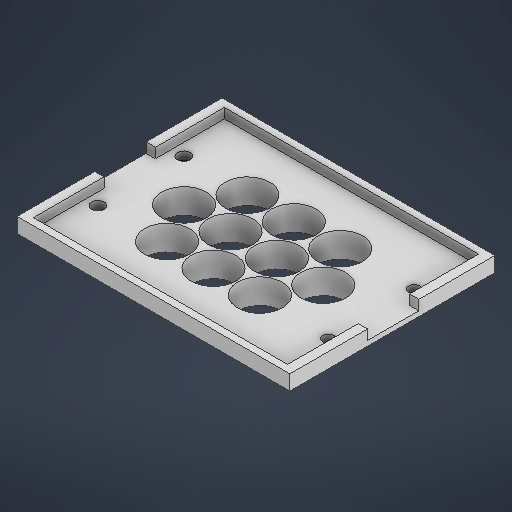
# Autodesk Inventor part: CELLCASE26650
Saved by Autodesk Inventor 2025.2 (Build 292293000, 293)
## iProperties
Created: 2025-01-16
Part Number: CELLCASE26650
Material: Generic
Document SubType Name: Modeling
Designer: cbast
Density: 1 g/cm^3
Appearance: Default
Author: cbast
## iProperties of the stored document CELLCASE26650_3DPrint.ipt
Created: 2025-01-31
Part Number: CELLCASE26650_3DPrint
Material: Generic
Document SubType Name: Modeling
Designer: cbast
Density: 1 g/cm^3
Appearance: Default
Author: cbast
Autodesk Inventor part; units mm, degrees
ref_plane "YZ Plane" through (0, 0, 0) normal (1, 0, 0) x (0, 1, 0)
ref_plane "XZ Plane" through (0, 0, 0) normal (0, 1, 0) x (-1, 0, 0)
ref_plane "XY Plane" through (0, 0, 0) normal (0, 0, 1) x (1, 0, 0)
sketch "Sketch1" plane through (0, 0, 0) normal (0, 1, 0) x (-1, 0, 0)
  circle A0 centre (0, 0) radius 13.5
  circle A1 centre (0, 0) radius 14.5 construction
  circle A2 centre (28, 0) radius 13.5
  circle A3 centre (28, 0) radius 14.5 construction
  circle A4 centre (56, 0) radius 13.5
  circle A5 centre (56, 0) radius 14.5 construction
  circle A6 centre (84, 0) radius 13.5
  circle A7 centre (84, 0) radius 14.5 construction
  circle A8 centre (14, 24.2487) radius 13.5
  circle A9 centre (42, 24.2487) radius 13.5
  circle A10 centre (70, 24.2487) radius 13.5
  circle A11 centre (70, -24.2487) radius 13.5
  circle A12 centre (42, -24.2487) radius 13.5
  circle A13 centre (14, -24.2487) radius 13.5
  line L0 (84, 0) -> (56, 0) construction
  circle A14 centre (14, 24.2487) radius 14.5 construction
  circle A15 centre (42, 24.2487) radius 14.5 construction
  circle A16 centre (70, 24.2487) radius 14.5 construction
  circle A17 centre (70, -24.2487) radius 14.5 construction
  circle A18 centre (42, -24.2487) radius 14.5 construction
  circle A19 centre (14, -24.2487) radius 14.5 construction
  circle A20 centre (0, 0) radius 15.5 construction
  circle A21 centre (14, 24.2487) radius 15.5 construction
  circle A22 centre (42, 24.2487) radius 15.5 construction
  circle A23 centre (70, 24.2487) radius 15.5 construction
  circle A24 centre (70, -24.2487) radius 15.5 construction
  circle A25 centre (42, -24.2487) radius 15.5 construction
  circle A26 centre (14, -24.2487) radius 15.5 construction
  arc A27 (1.2391, 15.4504) -> (1.2391, -15.4504) centre (0, 0) ccw
  arc A28 (28, 30.9008) -> (1.2391, 15.4504) centre (14, 24.2487) ccw
  arc A29 (56, 30.9008) -> (28, 30.9008) centre (42, 24.2487) ccw
  line L1 (70, 24.2487) -> (14, 24.2487) construction
  line L2 (14, 24.2487) -> (14, -24.2487) construction
  line L3 (14, -24.2487) -> (70, -24.2487) construction
  line L4 (70, -24.2487) -> (70, 24.2487) construction
  circle A30 centre (84, 0) radius 15.5 construction
  arc A31 (82.7609, 15.4504) -> (56, 30.9008) centre (70, 24.2487) ccw
  arc A32 (82.7609, -15.4504) -> (82.7609, 15.4504) centre (84, 0) ccw
  arc A33 (56, -30.9008) -> (82.7609, -15.4504) centre (70, -24.2487) ccw
  arc A34 (28, -30.9008) -> (56, -30.9008) centre (42, -24.2487) ccw
  arc A35 (1.2391, -15.4504) -> (28, -30.9008) centre (14, -24.2487) ccw
  dimension "d0" = 27
  dimension "d1" = 29
  dimension "d2" = 27
  dimension "d3" = 29
  dimension "d4" = 27
  dimension "d5" = 29
  dimension "d6" = 27
  dimension "d7" = 29
  dimension "d8" = 27
  dimension "d9" = 27
  dimension "d10" = 27
  dimension "d11" = 27
  dimension "d12" = 27
  dimension "d13" = 27
  dimension "d14" = 29
  dimension "d15" = 29
  dimension "d16" = 29
  dimension "d17" = 29
  dimension "d18" = 29
  dimension "d19" = 29
  dimension "d20" = 31
  dimension "d21" = 31
  dimension "d22" = 31
  dimension "d23" = 31
  dimension "d24" = 31
  dimension "d25" = 31
  dimension "d26" = 31
  dimension "d27" = 31
  constraints: 36 centre point, 32 point on circle, 27 coincident, 15 tangent, 10 end point, 2 horizontal, 1 perpendicular
  measures "d0" diameter of A0
  measures "d1" diameter of A1
  measures "d2" diameter of A2
  measures "d3" diameter of A3
  measures "d4" diameter of A4
  measures "d5" diameter of A5
  measures "d6" diameter of A6
  measures "d7" diameter of A7
  measures "d8" diameter of A8
  measures "d9" diameter of A9
  measures "d10" diameter of A10
  measures "d11" diameter of A11
  measures "d12" diameter of A12
  measures "d13" diameter of A13
  measures "d14" diameter of A14
  measures "d15" diameter of A15
  measures "d16" diameter of A16
  measures "d17" diameter of A17
  measures "d18" diameter of A18
  measures "d19" diameter of A19
  measures "d20" diameter of A20
  measures "d21" diameter of A21
  measures "d22" diameter of A22
  measures "d23" diameter of A23
  measures "d24" diameter of A24
  measures "d25" diameter of A25
  measures "d26" diameter of A26
  measures "d27" diameter of A30
extrude "Extrusion1" add sketch "Sketch1" along normal blind 15
sketch "Sketch2" plane through (0, 15, 0) normal (0, 1, 0) x (1, 0, 0)
  arc A0 (-1.2391, 15.4504) -> (-28, 30.9008) centre (-14, 24.2487) ccw projected
  arc A1 (-28, 30.9008) -> (-56, 30.9008) centre (-42, 24.2487) ccw projected
  arc A2 (-56, 30.9008) -> (-82.7609, 15.4504) centre (-70, 24.2487) ccw projected
  arc A3 (-82.7609, 15.4504) -> (-82.7609, -15.4504) centre (-84, 0) ccw projected
  arc A4 (-82.7609, -15.4504) -> (-56, -30.9008) centre (-70, -24.2487) ccw projected
  arc A5 (-56, -30.9008) -> (-28, -30.9008) centre (-42, -24.2487) ccw projected
  arc A6 (-28, -30.9008) -> (-1.2391, -15.4504) centre (-14, -24.2487) ccw projected
  arc A7 (-1.2391, -15.4504) -> (-1.2391, 15.4504) centre (0, 0) ccw projected
  circle A8 centre (-14, 24.2487) radius 13.5 projected
  circle A9 centre (-42, 24.2487) radius 13.5 projected
  circle A10 centre (-70, 24.2487) radius 13.5 projected
  circle A11 centre (-70, -24.2487) radius 13.5 projected
  circle A12 centre (-42, -24.2487) radius 13.5 projected
  circle A13 centre (-14, -24.2487) radius 13.5 projected
  circle A14 centre (-84, 0) radius 13.5 projected
  circle A15 centre (-56, 0) radius 13.5 projected
  circle A16 centre (-28, 0) radius 13.5 projected
  circle A17 centre (0, 0) radius 13.5 projected
  line L0 (-116.8, -58.15) -> (36.6, -58.15)
  line L1 (36.6, -58.15) -> (36.6, 57.15)
  line L2 (36.6, 57.15) -> (-116.8, 57.15)
  line L3 (-116.8, 57.15) -> (-116.8, -58.15)
  line L4 (-116.8, -58.15) -> (36.6, 57.15) construction
  line L5 (36.6, -58.15) -> (-116.8, 57.15) construction
  arc A18 (-82.7609, 15.4504) -> (-82.7609, -15.4504) centre (-84, 0) ccw
  arc A19 (-56, 30.9008) -> (-82.7609, 15.4504) centre (-70, 24.2487) ccw
  arc A20 (-28, 30.9008) -> (-56, 30.9008) centre (-42, 24.2487) ccw
  arc A21 (-1.2391, 15.4504) -> (-28, 30.9008) centre (-14, 24.2487) ccw
  arc A22 (-1.2391, -15.4504) -> (-1.2391, 15.4504) centre (0, 0) ccw
  arc A23 (-28, -30.9008) -> (-1.2391, -15.4504) centre (-14, -24.2487) ccw
  arc A24 (-56, -30.9008) -> (-28, -30.9008) centre (-42, -24.2487) ccw
  arc A25 (-82.7609, -15.4504) -> (-56, -30.9008) centre (-70, -24.2487) ccw
  point P0 (-40.1, -0.5)
  dimension "d30" = 153.4
  dimension "d31" = 115.3
  constraints: 16 point on circle, 12 end point, 8 centre point, 8 coincident, 2 midpoint, 2 parallel, 1 horizontal, 1 perpendicular
  measures "d30" distance of L2.end L1.end
  measures "d31" distance of L1.end L0.end
extrude "Extrusion2" add sketch "Sketch2" against normal blind 5 contours L3 L2 L1 L0
sketch "Sketch3" plane through (0, 15, 0) normal (0, 1, 0) x (1, 0, 0)
  line L0 (36.6, -58.15) -> (36.6, 57.15) projected
  line L1 (36.6, 57.15) -> (-116.8, 57.15) projected
  line L2 (-116.8, 57.15) -> (-116.8, -58.15) projected
  line L3 (-116.8, -58.15) -> (36.6, -58.15) projected
  circle A0 centre (-14, 24.2487) radius 13.5 projected
  circle A1 centre (-42, 24.2487) radius 13.5 projected
  circle A2 centre (-70, 24.2487) radius 13.5 projected
  circle A3 centre (-70, -24.2487) radius 13.5 projected
  circle A4 centre (-42, -24.2487) radius 13.5 projected
  circle A5 centre (-14, -24.2487) radius 13.5 projected
  circle A6 centre (-84, 0) radius 13.5 projected
  circle A7 centre (-56, 0) radius 13.5 projected
  circle A8 centre (-28, 0) radius 13.5 projected
  circle A9 centre (0, 0) radius 13.5 projected
  line L4 (-122.402, -62.3606) -> (42.202, -62.3606)
  line L5 (42.202, -62.3606) -> (42.202, 61.3606)
  line L6 (42.202, 61.3606) -> (-122.402, 61.3606)
  line L7 (-122.402, 61.3606) -> (-122.402, -62.3606)
  line L8 (-122.402, -62.3606) -> (42.202, 61.3606) construction
  line L9 (42.202, -62.3606) -> (-122.402, 61.3606) construction
  line L10 (-116.8, -58.15) -> (36.6, -58.15)
  line L11 (36.6, -58.15) -> (36.6, 57.15)
  line L12 (36.6, 57.15) -> (-116.8, 57.15)
  line L13 (-116.8, 57.15) -> (-116.8, -58.15)
  line L14 (-116.8, -58.15) -> (36.6, 57.15) construction
  line L15 (36.6, -58.15) -> (-116.8, 57.15) construction
  point P0 (-40.1, -0.5)
  constraints: 24 end point, 4 midpoint, 4 parallel, 4 point on line, 2 horizontal, 2 perpendicular
extrude "Extrusion3" add sketch "Sketch3" along normal blind 6 and the other way blind 3 contours L7 L6 L5 L4
sketch "Sketch4" plane through (0, 15, 0) normal (0, 1, 0) x (1, 0, 0)
  line L0 (36.6, -58.15) -> (36.6, 57.15) construction
  line L1 (36.6, 57.15) -> (-116.8, 57.15) construction
  line L2 (-116.8, 57.15) -> (-116.8, -58.15) construction
  line L3 (-116.8, -58.15) -> (36.6, -58.15) construction
  circle A0 centre (-14, 24.2487) radius 13.5 construction
  circle A1 centre (-42, 24.2487) radius 13.5 construction
  circle A2 centre (-70, 24.2487) radius 13.5 construction
  circle A3 centre (-70, -24.2487) radius 13.5 construction
  circle A4 centre (-42, -24.2487) radius 13.5 construction
  circle A5 centre (-14, -24.2487) radius 13.5 construction
  circle A6 centre (-84, 0) radius 13.5 construction
  circle A7 centre (-56, 0) radius 13.5 construction
  circle A8 centre (-28, 0) radius 13.5 construction
  circle A9 centre (0, 0) radius 13.5 construction
  line L4 (-116.8, 57.15) -> (-109.572, 57.15) construction
  line L5 (-109.572, 57.15) -> (-109.572, 25.4) construction
  line L6 (-109.572, 25.4) -> (-116.8, 25.4) construction
  line L7 (-116.8, 25.4) -> (-116.8, 57.15) construction
  line L8 (36.6, 57.15) -> (29.372, 57.15) construction
  line L9 (29.372, 57.15) -> (29.372, 25.4) construction
  line L10 (29.372, 25.4) -> (36.6, 25.4) construction
  line L11 (36.6, 25.4) -> (36.6, 57.15) construction
  line L12 (36.6, -58.15) -> (29.372, -58.15) construction
  line L13 (29.372, -58.15) -> (29.372, -26.4) construction
  line L14 (29.372, -26.4) -> (36.6, -26.4) construction
  line L15 (36.6, -26.4) -> (36.6, -58.15) construction
  line L16 (-116.8, -58.15) -> (-109.572, -58.15) construction
  line L17 (-109.572, -58.15) -> (-109.572, -26.4) construction
  line L18 (-109.572, -26.4) -> (-116.8, -26.4) construction
  line L19 (-116.8, -26.4) -> (-116.8, -58.15) construction
  circle A10 centre (-109.572, 25.4) radius 3.865
  circle A11 centre (29.372, 25.4) radius 3.365
  circle A12 centre (29.372, -26.4) radius 3.365
  circle A13 centre (-109.572, -26.4) radius 3.865
  dimension "d42" = 31.75
  dimension "d43" = 7.228
  dimension "d44" = 31.75
  dimension "d45" = 7.228
  dimension "d46" = 7.228
  dimension "d47" = 31.75
  dimension "d48" = 31.75
  dimension "d49" = 7.228
  dimension "d50" = 7.73
  dimension "d51" = 6.73
  dimension "d52" = 6.73
  dimension "d55" = 7.73
  constraints: 32 end point, 8 parallel, 4 centre point, 4 coincident, 4 horizontal, 4 perpendicular, 4 point on line
  measures "d42" distance of L4.end L5.end
  measures "d43" distance of L5.end L6.end
  measures "d44" distance of L8.end L9.end
  measures "d45" distance of L9.end L10.end
  measures "d46" distance of L13.end L14.end
  measures "d47" distance of L12.end L13.end
  measures "d48" distance of L16.end L17.end
  measures "d49" distance of L17.end L18.end
  measures "d50" diameter of A10
  measures "d51" diameter of A11
  measures "d52" diameter of A12
  measures "d55" diameter of A13
extrude "Extrusion4" cut sketch "Sketch4" against normal through all
sketch "Sketch5" plane through (-122.402, 12, 62.3606) normal (-1, 0, 0) x (0, 0, 1)
  line L0 (-77.8606, -12) -> (-77.8606, -2) projected
  line L1 (-46.9102, -12) -> (-46.9102, -2) projected
  line L2 (-119.5106, 3) -> (-4.2106, 3) projected
  line L3 (-123.7212, 9) -> (0, 9) projected
  line L4 (-77.8606, 3) -> (-46.9102, 3)
  line L5 (-46.9102, 3) -> (-46.9102, 9)
  line L6 (-46.9102, 9) -> (-77.8606, 9)
  line L7 (-77.8606, 9) -> (-77.8606, 3)
  point P0 (-62.3606, -12)
  constraints: 8 end point, 2 parallel, 2 point on line, 1 horizontal, 1 perpendicular
extrude "Extrusion5" cut sketch "Sketch5" against normal through all
body "Solid1"
